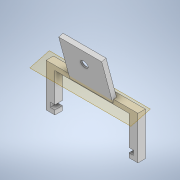
# Autodesk Inventor part: support_caméra
Saved by Autodesk Inventor 2020.2 (Build 242310000, 310)
## iProperties
Created: 2020-04-04
Part Number: support_caméra
Material: Générique
Document SubType Name: Modeling
Designer: anton
Density: 1 g/cm^3
Appearance: Par défaut
Author: anton
Autodesk Inventor part; units mm, degrees
ref_plane "YZ Plane" through (0, 0, 0) normal (1, 0, 0) x (0, 1, 0)
ref_plane "XZ Plane" through (0, 0, 0) normal (0, 1, 0) x (-1, 0, 0)
ref_plane "XY Plane" through (0, 0, 0) normal (0, 0, 1) x (1, 0, 0)
sketch "Esquisse1" plane through (0, 0, 0) normal (0, 0, 1) x (1, 0, 0)
  line L0 (-16.3902, 3.7398) -> (-19.3902, 3.7398)
  line L1 (-19.3902, 3.7398) -> (-19.3902, 0.7398)
  line L2 (-19.3902, 0.7398) -> (-16.3902, 0.7398)
  line L3 (-16.3902, 0.7398) -> (-16.3902, -2.2602)
  line L4 (-16.3902, -2.2602) -> (-22.3902, -2.2602)
  line L5 (-16.3902, 3.7398) -> (-16.3902, 23.7398)
  line L6 (33.6098, 23.7398) -> (33.6098, 3.7398)
  line L7 (33.6098, 3.7398) -> (36.6098, 3.7398)
  line L8 (36.6098, 3.7398) -> (36.6098, 0.7398)
  line L9 (36.6098, 0.7398) -> (33.6098, 0.7398)
  line L10 (33.6098, 0.7398) -> (33.6098, -2.2602)
  line L11 (33.6098, -2.2602) -> (39.6098, -2.2602)
  line L12 (-22.3902, 26.7398) -> (39.6098, 26.7398)
  line L13 (-16.3902, 23.7398) -> (33.6098, 23.7398)
  line L14 (-22.3902, 26.7398) -> (-22.3902, -2.2602)
  line L15 (39.6098, 26.7398) -> (39.6098, -2.2602)
  point P0 (0, 0)
  dimension "d0" = 56
  dimension "d1" = 3
  dimension "d2" = 3
  dimension "d3" = 3
  dimension "d4" = 3
  dimension "d5" = 20
  dimension "d6" = 20
  dimension "d7" = 50
  dimension "d8" = 3
  dimension "d9" = 6
  dimension "d10" = 6
  dimension "d11" = 3
  dimension "d12" = 3
  constraints: 32 end point, 7 perpendicular, 3 vertical, 2 point on line, 1 horizontal, 1 parallel
  measures "d0" distance between parallel lines of L8 L1
  measures "d1" distance of L0.end L1.end
  measures "d2" distance of L7.end L8.end
  measures "d3" distance of L2.end L3.end
  measures "d4" distance of L9.end L10.end
  measures "d5" distance of L6.start L6.end
  measures "d6" distance of L0.start L5.end
  measures "d7" distance between parallel lines of L6 L5
  measures "d8" distance of L0.start L0.end
  measures "d9" distance of L10.end L11.end
  measures "d10" distance of L3.end L4.end
  measures "d11" distance of L1.end L2.end
  measures "d12" distance between parallel lines of L12 L13
extrude "Extrusion1" add sketch "Esquisse1" along normal blind 5
ref_plane "Plan de construction1" through (39.6098, 26.7398, 5) normal (0, 0.9659258, 0.258819) x (-1, 0, 0)
sketch "Esquisse2" plane through (39.6098, 26.7398, 5) normal (0, 0.9659258, 0.258819) x (-1, 0, 0)
  line L0 (45.5, -2) -> (16.5, -2)
  line L1 (16.5, -2) -> (16.5, 1)
  line L2 (16.5, 1) -> (45.5, 1)
  line L3 (45.5, 1) -> (45.5, -2)
  line L4 (0, 0) -> (62, 0) projected
  line L5 (0, -4.8296) -> (0, 0) projected
  point P0 (39.6098, 2.0912)
  dimension "d16" = 29
  dimension "d17" = 3
  dimension "d18" = 1
  dimension "d23" = 16.5
  constraints: 8 end point, 2 parallel, 1 horizontal, 1 perpendicular
  measures "d16" distance of L0.start L0.end
  measures "d17" distance of L2.end L0.start
  measures "d18" distance between parallel lines of L2 L4
  measures "d23" distance between parallel lines of L5 L1
extrude "Extrusion2" add sketch "Esquisse2" along normal blind 27 and the other way blind 2
sketch "Esquisse3" plane through (23.1098, 26.7398, 2.9294) normal (0, 0.258819, -0.9659258) x (-1, 0, 0)
  line L0 (2, 25.5359) -> (27, 25.5359)
  line L1 (27, 25.5359) -> (27, 2.5359)
  line L2 (27, 2.5359) -> (2, 2.5359)
  line L3 (2, 2.5359) -> (2, 25.5359)
  line L4 (0, 27.5359) -> (29, 27.5359) projected
  line L5 (29, 0) -> (29, 27.5359) projected
  line L6 (-28.9, 0.5359) -> (57.9, 0.5359) projected
  line L7 (0, 27.5359) -> (0, 0) projected
  point P0 (23.1098, -26.5869)
  dimension "d24" = 2
  dimension "d25" = 2
  dimension "d26" = 2
  dimension "d27" = 2
  constraints: 8 end point, 2 parallel, 1 horizontal, 1 perpendicular
  measures "d24" distance between parallel lines of L4 L0
  measures "d25" distance between parallel lines of L5 L1
  measures "d26" distance between parallel lines of L6 L2
  measures "d27" distance between parallel lines of L7 L3
extrude "Extrusion3" cut sketch "Esquisse3" against normal blind 2 contours L0 L1 L2 L3
sketch "Esquisse4" plane through (23.1098, 26.2222, 4.8613) normal (0, 0.258819, -0.9659258) x (-1, 0, 0)
  circle A0 centre (14.3745, 17.1752) radius 2.5
  point P0 (23.1098, -26.5869)
  dimension "d30" = 5
  constraints: 1 centre point
  measures "d30" diameter of A0
extrude "Extrusion4" cut sketch "Esquisse4" against normal blind 10
